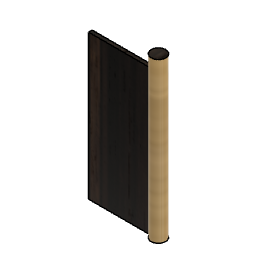
_4 per interior.698bebb2-d20f-4138-81ff-903649c77a47 (Autodesk Fusion 360 design; units mm, degrees)
Autodesk Fusion 360 part; units mm, degrees
note: some values were not read from the file. Set by a fixed rule: which face or edge a step refers to.
sketch "Sketch1" plane through (0, 0, 0.635) normal (0, 0, -1) x (1, 0, 0)
  circle A0 centre (0, 0) radius 6.35
  line L0 (0, 0) -> (-63.0682, 0)
  line L1 (-6.231, 1.5875) -> (-59.809, 1.5875)
  line L2 (-59.809, 1.5875) -> (-59.809, -1.5875)
  line L3 (-59.809, -1.5875) -> (-6.231, -1.5875)
  line L4 (-6.231, -1.5875) -> (-6.231, 1.5875)
  line L5 (-6.231, 1.5875) -> (-59.809, -1.5875) construction
  line L6 (-59.809, 1.5875) -> (-6.231, -1.5875) construction
  point P0 (-33.02, 0)
  dimension "d3" = 12.7
  dimension "d4" = 63.0682
  dimension "d5" = 3.175
  constraint coincident A0.centre L0.start
  constraint horizontal L0
  constraint horizontal L1
  constraint perpendicular L1 L2
  constraint parallel L1 L3
  constraint parallel L2 L4
  constraint coincident L5 P0
  constraint coincident L6 P0
  constraint coincident L0 P0
  measures "d3" diameter of A0
  measures "d4" distance of A0.centre L0.end
  measures "d5" distance of L1.end L2.end
extrude "Extrude4" add sketch "Sketch1" along normal blind 127 contours A0 L4 | A0 L0 L1 L2 L4 | A0 L0 L2 L3 L4
extrude "Extrude5" add 1 faces at (-1.3187, -3.4497, 0.635) along direction (0, 0, 1) blind 12.7
